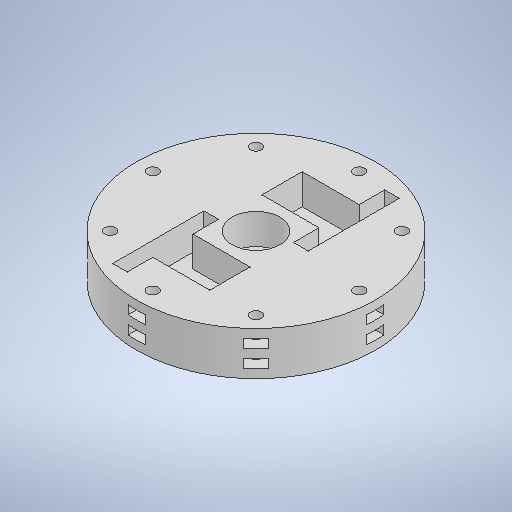
# Autodesk Inventor part: SCARA swivel base - top
Saved by Autodesk Inventor 2025.2 (Build 292293000, 293)
## iProperties
Created: 2025-01-25
Part Number: SCARA swivel base - top
Material: Generic
Document SubType Name: Modeling
Designer: caomi
Density: 1 g/cm^3
Appearance: Default
Author: caomi
Autodesk Inventor part; units mm, degrees
ref_plane "YZ Plane" through (0, 0, 0) normal (1, 0, 0) x (0, 1, 0)
ref_plane "XZ Plane" through (0, 0, 0) normal (0, 1, 0) x (-1, 0, 0)
ref_plane "XY Plane" through (0, 0, 0) normal (0, 0, 1) x (1, 0, 0)
sketch "Sketch1" plane through (0, 0, 0) normal (0, 1, 0) x (-1, 0, 0)
  circle A0 centre (0, 0) radius 55
  line L0 (20, 46) -> (20, 4)
  line L1 (20, 4) -> (13.25, 4)
  line L2 (13.25, 4) -> (13.25, 15.75)
  line L3 (13.25, 15.75) -> (-13, 15.75)
  line L4 (-13, 15.75) -> (-13, 34.25)
  line L5 (-13, 34.25) -> (13.25, 34.25)
  line L6 (13.25, 34.25) -> (13.25, 46)
  line L7 (13.25, 46) -> (20, 46)
  line L8 (45.5655, 25) -> (-15.5039, 25) construction
  line L9 (0, -77) -> (0, 77) projected
  line L10 (-20, -4) -> (-20, -46)
  line L11 (-20, -46) -> (-13.25, -46)
  line L12 (-13.25, -46) -> (-13.25, -34.25)
  line L13 (-13.25, -34.25) -> (13, -34.25)
  line L14 (13, -34.25) -> (13, -15.75)
  line L15 (13, -15.75) -> (-13.25, -15.75)
  line L16 (-13.25, -15.75) -> (-13.25, -4)
  line L17 (-13.25, -4) -> (-20, -4)
  line L18 (19.1191, -25) -> (-71.9329, -25) construction
  line L19 (80.3866, 0) -> (-97.3195, 0) projected
  circle A1 centre (0, 0) radius 11
  circle A2 centre (0, 0) radius 4
  point P0 (0, -4.3524)
  point P1 (0, -25)
  point P2 (0, 25)
  dimension "d0" = 6.75
  dimension "d1" = 18.5
  dimension "d2" = 110
  dimension "d3" = 33
  dimension "d4" = 42
  dimension "d12" = 22
  dimension "d24" = 20
  dimension "d25" = 20
  dimension "d26" = 50
  dimension "d50" = 8
  constraints: 36 end point, 10 perpendicular, 7 point on line, 4 horizontal, 4 parallel, 3 centre point, 2 coincident, 2 vertical, 1 midpoint, 1 vertical alignment, 6 other
  measures "d0" distance between parallel lines of L2 L0
  measures "d1" distance of L3.end L4.end
  measures "d2" diameter of A0
  measures "d3" distance between parallel lines of L0 L4
  measures "d4" distance between parallel lines of L1 L7
  measures "d12" diameter of A1
  measures "d24" distance from line of point (0, -25) L10
  measures "d25" distance from line of point (0, 25) L0
  measures "d26" distance of point (0, 25) point (0, -25)
  measures "d50" diameter of A2
extrude "Extrusion1" add sketch "Sketch1" along normal blind 20 contours L19 A1 L9 L3 L2 L1 L0 L7 L6 L5 A0 | A0 L9 L13 L14 L15 A1 L19 | L9 L5 L4 L3 A1 L19 A0 | A0 L19 A1 L9 L15 L16 L17 L10 L11 L12 L13
extrude "Extrusion2" add sketch "Sketch1" along normal blind 6 contours L9 L3 L4 L5 | L5 L6 L7 L0 L1 L2 L3 L9 | L13 L12 L11 L10 L17 L16 L15 L9 | L9 L15 L14 L13
extrude "Extrusion6" add sketch "Sketch1" along normal up to surface (6 mm away) contours A1 L9 A2 L19 | L19 A2 L9 A1 | A2 L9 L19 | L19 L9 A2 | L9 A2 L19 A1 | A1 L19 A2 L9 | L19 A2 L9 | L9 A2 L19
sketch "Sketch4" plane through (0, 20, 0) normal (0, 1, 0) x (1, 0, 0)
  circle A0 centre (-47.5, 0) radius 2.5
  line L0 (-58.18, 4) -> (-45.4144, 4)
  line L1 (-45.4144, 4) -> (-43.105, 0)
  line L2 (-43.105, 0) -> (-45.4144, -4)
  line L3 (-45.4144, -4) -> (-58.18, -4)
  line L4 (-58.18, -4) -> (-58.18, 4)
  line L5 (0, 0) -> (-69.9236, 0) construction
  circle A1 centre (0, 0) radius 55 projected
  dimension "d32" = 5
  dimension "d33" = 60
  dimension "d34" = 8
  dimension "d35" = 4.395
  dimension "d44" = 47.5
  constraints: 12 end point, 2 horizontal, 1 centre point, 1 parallel, 1 point on line, 1 vertical, 2 other
  measures "d32" diameter of A0
  measures "d33" angle of L1 L5
  measures "d34" distance between parallel lines of L0 L3
  measures "d35" distance of L1.end A0.centre
  measures "d44" distance of A0.centre A1.centre
ref_plane "Work Plane2" through (0, 14, 0) normal (0, 1, 0) x (1, 0, 0)
ref_plane "Work Plane3" through (0, 6, 0) normal (0, 1, 0) x (1, 0, 0)
extrude "Extrusion4" cut sketch "Sketch4" along normal mid plane 4 from surface at -14 contours A0 | L0 A1 L3 L4 | L0 L1 L2 L3 A1 picked at (-49.5518, 3.4458)
extrude "Extrusion5" cut sketch "Sketch4" along normal mid plane 4 from surface at -6 contours A0 | L0 A1 L3 L4 | L0 L1 L2 L3 A1 picked at (-49.5518, 3.4458)
extrude "Extrusion7" cut sketch "Sketch4" against normal up to surface (20 mm away) contours A0
pattern_circular "Circular Pattern1" count 8 over 360 about axis through (0, 0, 0) along (0, 1, 0) of "Extrusion5", "Extrusion4", "Extrusion7"
equation "\"d24\" = d23"
equation "\"d23\" = 20"
body "Solid1"
